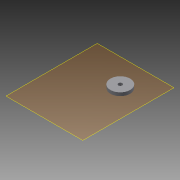
# Autodesk Inventor part: spacer
Saved by Autodesk Inventor 2014 (Build 180170000, 170)
## iProperties
Created: 2014-03-06
Part Number: spacer
Material: 常规
Document SubType Name: Modeling
Designer: Keshuai
Density: 1 g/cm^3
Appearance: 默认
Author: Keshuai
Autodesk Inventor part; units mm, degrees
ref_plane "YZ Plane" through (0, 0, 0) normal (1, 0, 0) x (0, 1, 0)
ref_plane "XZ Plane" through (0, 0, 0) normal (0, 1, 0) x (-1, 0, 0)
ref_plane "XY Plane" through (0, 0, 0) normal (0, 0, 1) x (1, 0, 0)
ref_plane "工作平面1" through (0, 0, 0) normal (0, 0, 1) x (1, 0, 0)
sketch "草图2" plane through (0, 0, 0) normal (0, 0, 1) x (1, 0, 0)
  circle A0 centre (-10.2751, -46) radius 3.6 projected
  line L0 (17, -14) -> (17, -46) projected
  line L1 (17, -46) -> (-1, -46) projected
  line L2 (-1, -46) -> (-1, -14) projected
  line L3 (-1, -14) -> (17, -14) projected
  line L4 (48, 25.5) -> (41.2, 25.5) projected
  line L5 (41.2, 25.5) -> (41.2, 23.75) projected
  line L6 (41.2, 23.75) -> (38.8, 23.75) projected
  line L7 (38.8, 23.75) -> (38.8, 25.5) projected
  line L8 (38.8, 25.5) -> (36, 25.5) projected
  line L9 (36, 25.5) -> (36, 28.5) projected
  line L10 (36, 28.5) -> (38.8, 28.5) projected
  line L11 (38.8, 28.5) -> (38.8, 30.25) projected
  line L12 (38.8, 30.25) -> (41.2, 30.25) projected
  line L13 (41.2, 30.25) -> (41.2, 28.5) projected
  line L14 (41.2, 28.5) -> (48, 28.5) projected
  line L15 (48, 28.5) -> (48, 42) projected
  line L16 (48, 42) -> (53, 42) projected
  line L17 (53, 42) -> (53, 63) projected
  line L18 (53, 63) -> (15, 63) projected
  line L19 (15, 58) -> (15, 63) projected
  line L20 (1.5, 58) -> (15, 58) projected
  line L21 (1.5, 58) -> (1.5, 51.2) projected
  line L22 (1.5, 51.2) -> (3.25, 51.2) projected
  line L23 (3.25, 51.2) -> (3.25, 48.8) projected
  line L24 (3.25, 48.8) -> (1.5, 48.8) projected
  line L25 (1.5, 48.8) -> (1.5, 46) projected
  line L26 (1.5, 46) -> (-1.5, 46) projected
  line L27 (-1.5, 46) -> (-1.5, 48.8) projected
  line L28 (-1.5, 48.8) -> (-3.25, 48.8) projected
  line L29 (-3.25, 48.8) -> (-3.25, 51.2) projected
  line L30 (-3.25, 51.2) -> (-1.5, 51.2) projected
  line L31 (-1.5, 51.2) -> (-1.5, 58) projected
  line L32 (-15, 58) -> (-1.5, 58) projected
  line L33 (-15, 58) -> (-15, 63) projected
  line L34 (-15, 63) -> (-53, 63) projected
  line L35 (-53, 63) -> (-53, 42) projected
  line L36 (-48, 42) -> (-53, 42) projected
  line L37 (-48, 28.5) -> (-48, 42) projected
  line L38 (-48, 28.5) -> (-41.2, 28.5) projected
  line L39 (-41.2, 28.5) -> (-41.2, 30.25) projected
  line L40 (-41.2, 30.25) -> (-38.8, 30.25) projected
  line L41 (-38.8, 30.25) -> (-38.8, 28.5) projected
  line L42 (-38.8, 28.5) -> (-36, 28.5) projected
  line L43 (-36, 28.5) -> (-36, 25.5) projected
  line L44 (-36, 25.5) -> (-38.8, 25.5) projected
  line L45 (-38.8, 25.5) -> (-38.8, 23.75) projected
  line L46 (-38.8, 23.75) -> (-41.2, 23.75) projected
  line L47 (-41.2, 23.75) -> (-41.2, 25.5) projected
  line L48 (-41.2, 25.5) -> (-48, 25.5) projected
  line L49 (-48, 12) -> (-48, 25.5) projected
  line L50 (-48, 12) -> (-53, 12) projected
  line L51 (-53, 12) -> (-53, -8) projected
  line L52 (-48, -8) -> (-53, -8) projected
  line L53 (-48, -21.5) -> (-48, -8) projected
  line L54 (-48, -21.5) -> (-41.2, -21.5) projected
  line L55 (-41.2, -21.5) -> (-41.2, -19.75) projected
  line L56 (-41.2, -19.75) -> (-38.8, -19.75) projected
  line L57 (-38.8, -19.75) -> (-38.8, -21.5) projected
  line L58 (-38.8, -21.5) -> (-36, -21.5) projected
  line L59 (-36, -21.5) -> (-36, -24.5) projected
  line L60 (-36, -24.5) -> (-38.8, -24.5) projected
  line L61 (-38.8, -24.5) -> (-38.8, -26.25) projected
  line L62 (-38.8, -26.25) -> (-41.2, -26.25) projected
  line L63 (-41.2, -26.25) -> (-41.2, -24.5) projected
  line L64 (-41.2, -24.5) -> (-48, -24.5) projected
  line L65 (-48, -38) -> (-48, -24.5) projected
  line L66 (-48, -38) -> (-53, -38) projected
  line L67 (-53, -38) -> (-53, -63) projected
  line L68 (-53, -63) -> (-15, -63) projected
  line L69 (-15, -58) -> (-15, -63) projected
  line L70 (-15, -58) -> (15, -58) projected
  line L71 (15, -58) -> (15, -63) projected
  line L72 (15, -63) -> (53, -63) projected
  line L73 (53, -63) -> (53, -38) projected
  line L74 (48, -38) -> (53, -38) projected
  line L75 (48, -38) -> (48, -24.5) projected
  line L76 (48, -24.5) -> (41.2, -24.5) projected
  line L77 (41.2, -24.5) -> (41.2, -26.25) projected
  line L78 (41.2, -26.25) -> (38.8, -26.25) projected
  line L79 (38.8, -26.25) -> (38.8, -24.5) projected
  line L80 (38.8, -24.5) -> (36, -24.5) projected
  line L81 (36, -24.5) -> (36, -21.5) projected
  line L82 (36, -21.5) -> (38.8, -21.5) projected
  line L83 (38.8, -21.5) -> (38.8, -19.75) projected
  line L84 (38.8, -19.75) -> (41.2, -19.75) projected
  line L85 (41.2, -19.75) -> (41.2, -21.5) projected
  line L86 (41.2, -21.5) -> (48, -21.5) projected
  line L87 (48, -21.5) -> (48, -8) projected
  line L88 (48, -8) -> (53, -8) projected
  line L89 (53, -8) -> (53, 12) projected
  line L90 (48, 12) -> (53, 12) projected
  line L91 (48, 12) -> (48, 25.5) projected
  circle A1 centre (18, 28) radius 3 projected
  line L92 (28, -10) -> (28, -5) projected
  line L93 (28, -5) -> (43, -5) projected
  line L94 (43, -5) -> (43, -10) projected
  line L95 (43, -10) -> (28, -10) projected
  line L96 (-2, -10) -> (-2, -5) projected
  line L97 (-2, -5) -> (13, -5) projected
  line L98 (13, -5) -> (13, -10) projected
  line L99 (13, -10) -> (-2, -10) projected
  line L100 (-20, 17) -> (-20, 32) projected
  line L101 (-20, 32) -> (-15, 32) projected
  line L102 (-15, 32) -> (-15, 17) projected
  line L103 (-15, 17) -> (-20, 17) projected
  line L104 (-20, -13) -> (-20, 2) projected
  line L105 (-20, 2) -> (-15, 2) projected
  line L106 (-15, 2) -> (-15, -13) projected
  line L107 (-15, -13) -> (-20, -13) projected
  line L108 (-23, 42) -> (-23, 37) projected
  line L109 (-23, 37) -> (-43, 37) projected
  line L110 (-43, 37) -> (-43, 42) projected
  line L111 (-43, 42) -> (-23, 42) projected
  circle A2 centre (18, 28) radius 15
  point P0 (0, 0)
  dimension "d0" = 30
  constraints: 1 centre point, 1 coincident
  measures "d0" diameter of A2
extrude "拉伸1" add sketch "草图2" along normal blind 5 contours A2
